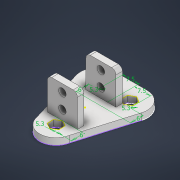
# Autodesk Inventor part: Stationary bracket V3
Saved by Autodesk Inventor 2022 (Build 260153000, 153)
## iProperties
Created: 2022-01-30
Part Number: Stationary bracket V3
Material: Generic
Document SubType Name: Modeling
Designer: izack
Density: 1 g/cm^3
Appearance: Default
Author: izack
## iProperties of the stored document Stationary Bracket_3DPrint.ipt
Part Number: Stationary Bracket_3DPrint
Material: Generic
Document SubType Name: Modeling
Designer: izack
Appearance: Default
Author: izack
Autodesk Inventor part; units mm, degrees
ref_plane "YZ Plane" through (0, 0, 0) normal (1, 0, 0) x (0, 1, 0)
ref_plane "XZ Plane" through (0, 0, 0) normal (0, 1, 0) x (-1, 0, 0)
ref_plane "XY Plane" through (0, 0, 0) normal (0, 0, 1) x (1, 0, 0)
sketch "Sketch1" plane through (0, 0, 0) normal (0, 1, 0) x (-1, 0, 0)
  line L0 (-7, 10.5) -> (7, 10.5)
  line L1 (7, 10.5) -> (7, -10.5)
  line L2 (7, -10.5) -> (-7, -10.5)
  line L3 (-7, -10.5) -> (-7, 10.5)
  line L4 (-7, 10.5) -> (7, -10.5) construction
  line L5 (7, 10.5) -> (-7, -10.5) construction
  line L6 (-7, 7.5) -> (7, 7.5)
  line L7 (7, 7.5) -> (7, -7.5)
  line L8 (7, -7.5) -> (-7, -7.5)
  line L9 (-7, -7.5) -> (-7, 7.5)
  line L10 (-7, 7.5) -> (7, -7.5) construction
  line L11 (7, 7.5) -> (-7, -7.5) construction
  line L12 (7, 0) -> (-7, 0) construction
  circle A0 centre (3.5, 0) radius 1.25
  circle A1 centre (-3.5, 0) radius 1.25
  point P0 (0, 0)
  dimension "d0" = 14
  dimension "d1" = 21
  dimension "d2" = 15
  dimension "d3" = 2.5
  dimension "d4" = 2.5
  dimension "d5" = 3.5
  dimension "d6" = 3.5
  constraints: 26 end point, 6 midpoint, 4 parallel, 3 point on line, 2 centre point, 2 horizontal, 2 perpendicular
  measures "d0" distance of L1.end L2.end
  measures "d1" distance of L0.end L1.end
  measures "d2" distance of L6.end L7.end
  measures "d3" diameter of A0
  measures "d4" diameter of A1
  measures "d5" distance from line of L1 A0.centre
  measures "d6" distance from line of L3 A1.centre
extrude "Extrusion1" add sketch "Sketch1" along normal blind 3
sketch "Sketch2" plane through (0, 0, 0) normal (0, -1, 0) x (1, 0, 0)
  line L0 (7, -10.5) -> (-7, -10.5) projected
  line L1 (7, 10.5) -> (7, -10.5) projected
  line L2 (-7, -10.5) -> (7, -10.5)
  line L3 (7, -10.5) -> (7, -7.5)
  line L4 (7, -7.5) -> (-7, -7.5)
  line L5 (-7, -7.5) -> (-7, -10.5)
  line L6 (-7, 10.5) -> (7, 10.5) projected
  line L7 (-7, 10.5) -> (7, 10.5)
  line L8 (7, 10.5) -> (7, 7.5)
  line L9 (7, 7.5) -> (-7, 7.5)
  line L10 (-7, 7.5) -> (-7, 10.5)
  point P0 (0, 0)
  dimension "d9" = 3
  dimension "d10" = 3
  constraints: 16 end point, 4 parallel, 2 horizontal, 2 perpendicular, 2 point on line
  measures "d9" distance of L3.end L2.end
  measures "d10" distance of L7.end L8.end
extrude "Extrusion2" add sketch "Sketch2" along normal blind 18
sketch "Sketch3" plane through (-7, 3, 10.5) normal (0, 0, 1) x (1, 0, 0)
  line L0 (14, -3) -> (0, -3) projected
  line L1 (0, -3) -> (14, -3)
  line L2 (0, -3) -> (0, -21) construction
  line L3 (0, -6.5) -> (14, -6.5) construction
  circle A0 centre (7, -13.5) radius 1.75
  circle A1 centre (7, -6.5) radius 1.75
  line L4 (14, -21) -> (14, 0) projected
  line L5 (7, -3) -> (7, -16.789) construction
  dimension "d14" = 3.5
  dimension "d15" = 3.5
  dimension "d32" = 3.5
  dimension "d33" = 7
  constraints: 6 end point, 3 point on line, 2 centre point, 1 collinear, 1 horizontal, 1 midpoint, 1 vertical
  measures "d14" diameter of A0
  measures "d15" diameter of A1
  measures "d32" distance from line of A1.centre L0
  measures "d33" distance of A1.centre A0.centre
extrude "Extrusion3" cut sketch "Sketch3" against normal through all
sketch "Sketch4" plane through (-7, 0, -7.5) normal (0, 0, 1) x (1, 0, 0)
  line L0 (0, 0) -> (0, -18) projected
  line L1 (14, 0) -> (14, -18) projected
  line L2 (0, -18) -> (14, -18)
  line L3 (14, -18) -> (14, -15)
  line L4 (14, -15) -> (0, -15)
  line L5 (0, -15) -> (0, -18)
  point P0 (7, 0)
  point P1 (0, -15)
  dimension "d20" = 3
  constraints: 8 end point, 2 parallel, 1 horizontal, 1 perpendicular, 1 point on line
  measures "d20" distance of L3.end L2.end
extrude "Extrusion4" add sketch "Sketch4" along normal up to surface (15 mm away)
sketch "Sketch5" plane through (0, -18, 0) normal (0, -1, 0) x (1, 0, 0)
  circle A0 centre (7.5, -13.5) radius 2.65
  circle A1 centre (0, 13.5) radius 2.65
  line L0 (7, 10.5) -> (-7, 10.5) projected
  line L1 (-7, -10.5) -> (7, -10.5) projected
  line L2 (-7, 10.5) -> (-7, -10.5) projected
  line L3 (-7, 10.5) -> (7, 10.5)
  line L4 (-7, -10.5) -> (7, -10.5)
  line L5 (-1.75, 10.5) -> (1.75, 10.5) construction
  line L6 (0, 10.5) -> (0, -10.5) construction
  line L7 (7, -10.5) -> (-7, -10.5) construction
  circle A2 centre (-7.5, -13.5) radius 2.65
  line L8 (-7, 10.5) -> (7, 10.5) projected
  circle A3 centre (0, 13.5) radius 7.6158
  circle A4 centre (7.5, -13.5) radius 8.0777
  circle A5 centre (-7.5, -13.5) radius 8.0777
  line L9 (-7.5, 14.8229) -> (-15.2423, -11.1962)
  line L10 (-7.5, -21.5777) -> (7.5, -21.5777)
  line L11 (15.2423, -11.1962) -> (7.5, 14.8229)
  line L12 (-4.85, -15.03) -> (-7.5, -16.56)
  line L13 (-7.5, -16.56) -> (-10.15, -15.03)
  line L14 (-10.15, -15.03) -> (-10.15, -11.97)
  line L15 (-10.15, -11.97) -> (-7.5, -10.44)
  line L16 (-7.5, -10.44) -> (-4.85, -11.97)
  line L17 (-4.85, -11.97) -> (-4.85, -15.03)
  line L18 (10.15, -15.03) -> (7.5, -16.56)
  line L19 (7.5, -16.56) -> (4.85, -15.03)
  line L20 (4.85, -15.03) -> (4.85, -11.97)
  line L21 (4.85, -11.97) -> (7.5, -10.44)
  line L22 (7.5, -10.44) -> (10.15, -11.97)
  line L23 (10.15, -11.97) -> (10.15, -15.03)
  line L24 (2.5773, 11.8505) -> (-0.1399, 10.4432)
  line L25 (-0.1399, 10.4432) -> (-2.7172, 12.0927)
  line L26 (-2.7172, 12.0927) -> (-2.5773, 15.1495)
  line L27 (-2.5773, 15.1495) -> (0.1399, 16.5568)
  line L28 (0.1399, 16.5568) -> (2.7172, 14.9073)
  line L29 (2.7172, 14.9073) -> (2.5773, 11.8505)
  point P0 (0, 0)
  point P1 (-7, -7.5)
  point P2 (-7, 7.5)
  point P3 (0, -13.5)
  point P4 (4.85, -13.5)
  point P5 (-2.65, 13.5)
  point P6 (-10.1305, -13.8206)
  point P7 (0, -16.5)
  point P8 (-2.413, 10.5)
  point P9 (2.413, 10.5)
  point P10 (-7, -9.6826)
  point P11 (-5.087, -10.5)
  point P12 (-4.85, -13.5)
  point P13 (10.15, -13.5)
  point P14 (2.6472, 13.3789)
  point P15 (-0.2285, 10.5)
  point P16 (-0.0303, 10.5)
  point P17 (0, -10.5)
  point P18 (0, -10.5)
  point P19 (-7, -5.4377)
  dimension "d23" = 5.3
  dimension "d24" = 5.3
  dimension "d25" = 6
  dimension "d26" = 6
  dimension "d34" = 7.5
  dimension "d35" = 5.3
  dimension "d36" = 7.5
  dimension "d37" = 6
  constraints: 48 end point, 15 point on circle, 7 coincident, 6 centre point, 5 midpoint, 2 equal length, 2 tangent, 1 horizontal, 39 other
  measures "d23" diameter of A0
  measures "d24" diameter of A1
  measures "d25" vertical distance of point (-7, -7.5) A0.centre
  measures "d26" vertical distance of A1.centre point (-7, 7.5)
  measures "d34" distance from line of L6 A0.centre
  measures "d35" diameter of A2
  measures "d36" distance from line of L6 A2.centre
  measures "d37" vertical distance of point (-7, -7.5) A2.centre
extrude "Extrusion5" add sketch "Sketch5" against normal blind 3 contours L28 L27 L26 L25 L0 A3 L24 L29 | A3 L11 A4 A5 L2 | L2 A5 L9 A3 | L2 L1 A4 A5 | A5 A4 | A4 A5 | A4 L10 A5
sketch "Sketch6" plane through (0, 3, 0) normal (0, 1, 0) x (1, 0, 0)
  line L0 (-7, 10.5) -> (-7, -10.5) projected
  line L1 (-7, -10.5) -> (7, -10.5) projected
  line L2 (-7, -10.5) -> (7, -10.5) projected
  line L3 (7, -10.5) -> (7, 10.5) projected
  line L4 (7, 10.5) -> (-7, 10.5) projected
  line L5 (-7, 10.5) -> (-7, -10.5) projected
  circle A0 centre (3.5, 0) radius 1.25 projected
  circle A1 centre (-3.5, 0) radius 1.25 projected
  point P0 (0, 0)
extrude "Extrusion6" cut sketch "Sketch6" against normal up to surface (3 mm away)
fillet "Fillet1" radius 2 4 edges at (-7, 0, -9) (7, 0, -9) (-7, 0, 9) (7, 0, 9)
sketch "Sketch10" plane through (0, -15, 13.5) normal (0, 1, 0) x (1, 0, 0)
  line L0 (-10.15, 25.47) -> (-10.15, 28.53) projected
  line L1 (-10.15, 28.53) -> (-7.5, 30.06) projected
  line L2 (-7.5, 30.06) -> (-4.85, 28.53) projected
  line L3 (-4.85, 28.53) -> (-4.85, 25.47) projected
  line L4 (-4.85, 25.47) -> (-7.5, 23.94) projected
  line L5 (-7.5, 23.94) -> (-10.15, 25.47) projected
  line L6 (4.85, 28.53) -> (7.5, 30.06) projected
  line L7 (4.85, 25.47) -> (4.85, 28.53) projected
  line L8 (7.5, 23.94) -> (4.85, 25.47) projected
  line L9 (10.15, 25.47) -> (7.5, 23.94) projected
  line L10 (10.15, 28.53) -> (10.15, 25.47) projected
  line L11 (7.5, 30.06) -> (10.15, 28.53) projected
  line L12 (2.5773, 1.6495) -> (2.7172, -1.4073) projected
  line L13 (-0.0303, 3) -> (2.5773, 1.6495) projected
  line L14 (-2.7172, 1.4073) -> (-0.2285, 3) projected
  line L15 (-2.5773, -1.6495) -> (-2.7172, 1.4073) projected
  line L16 (0.1399, -3.0568) -> (-2.5773, -1.6495) projected
  line L17 (2.7172, -1.4073) -> (0.1399, -3.0568) projected
  point P0 (0, 13.5)
body "Solid1"
